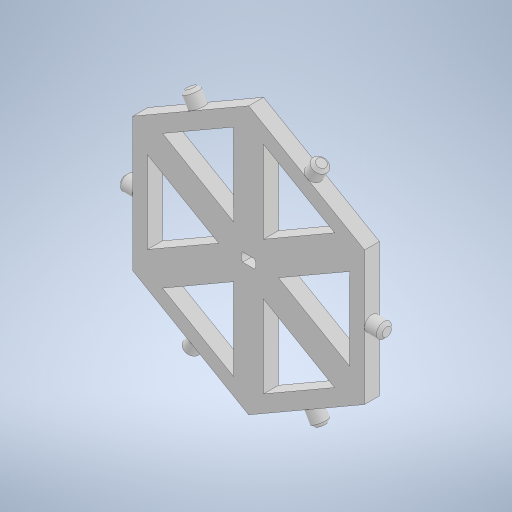
# Autodesk Inventor part: inner_case_bottom
Saved by Autodesk Inventor 2024 (Build 280153000, 153)
## iProperties
Created: 2024-03-18
Part Number: inner_case_bottom
Material: 일반
Document SubType Name: Modeling
Designer: SSAFY
Density: 1 g/cm^3
Appearance: 기본값
Author: SSAFY
Autodesk Inventor part; units mm, degrees
ref_plane "YZ Plane" through (0, 0, 0) normal (1, 0, 0) x (0, 1, 0)
ref_plane "XZ Plane" through (0, 0, 0) normal (0, 1, 0) x (-1, 0, 0)
ref_plane "XY Plane" through (0, 0, 0) normal (0, 0, 1) x (1, 0, 0)
sketch "스케치1" plane through (0, 0, 0) normal (0, 0, 1) x (1, 0, 0)
  line L0 (0.041, 45.0463) -> (39.005, 22.534)
  line L1 (39.005, 22.534) -> (38.9908, -22.466)
  line L2 (38.9908, -22.466) -> (0.0125, -44.9537)
  line L3 (0.0125, -44.9537) -> (-38.9515, -22.4414)
  line L4 (-38.9515, -22.4414) -> (-38.9373, 22.5586)
  line L5 (-38.9373, 22.5586) -> (0.041, 45.0463)
  line L6 (-38.9373, 22.5586) -> (0, 0)
  line L7 (0, 0) -> (-0.0392, 45.0926)
  line L8 (-5.0075, 8.6797) -> (-5.0316, 36.3473)
  line L9 (0.0143, -39.1802) -> (0.0341, -39.1916)
  line L10 (-28.9475, 22.5495) -> (-5.0075, 8.6797)
  line L11 (-28.9475, 22.5495) -> (-5.0316, 36.3473)
  line L12 (-0.0341, 39.2305) -> (0.0392, 39.2728)
  line L13 (5.0131, 8.6765) -> (28.9619, 22.5311)
  line L14 (5.0547, 36.3441) -> (28.9619, 22.5311)
  line L15 (5.0547, 36.3441) -> (5.0131, 8.6765)
  line L16 (10.0206, -0.0032) -> (33.9935, -13.8162)
  line L17 (34.0023, 13.7945) -> (33.9935, -13.8162)
  line L18 (34.0023, 13.7945) -> (10.0206, -0.0032)
  line L19 (5.0075, -8.6797) -> (5.0316, -36.3473)
  line L20 (28.9475, -22.5495) -> (5.0316, -36.3473)
  line L21 (28.9475, -22.5495) -> (5.0075, -8.6797)
  line L22 (-5.0131, -8.6765) -> (-28.9619, -22.5311)
  line L23 (-5.0547, -36.3441) -> (-28.9619, -22.5311)
  line L24 (-5.0547, -36.3441) -> (-5.0131, -8.6765)
  line L25 (-10.0206, 0.0032) -> (-33.9935, 13.8162)
  line L26 (-34.0023, -13.7945) -> (-33.9935, 13.8162)
  line L27 (-34.0023, -13.7945) -> (-10.0206, 0.0032)
  circle A0 centre (0, 0) radius 2.5
  line L28 (-2.0013, 1.4983) -> (1.9987, 1.5017)
  line L29 (-1.9987, -1.5017) -> (2.0013, -1.4983)
  dimension "d19" = 45
  dimension "d20" = 5
  dimension "d22" = 5
  dimension "d23" = 5
  dimension "d26" = 360
  dimension "d28" = 5
  dimension "d29" = 1.5
  dimension "d30" = 1.5
  constraints: 60 end point, 4 coincident, 4 point on circle, 3 point on line, 1 centre point, 1 parallel, 1 perpendicular, 41 other
  measures "d19" distance of L3.end L4.end
  measures "d20" distance between parallel lines of L7 L8
  measures "d22" distance between parallel lines of L11 L5
  measures "d23" distance between parallel lines of L6 L10
  measures "d28" diameter of A0
  measures "d29" distance from line of L28 L6.end
  measures "d30" distance from line of L29 point (0, 0)
extrude "돌출1" add sketch "스케치1" along normal blind 5 contours L0 L1 L2 L3 L4 L6 A0 L7 L5 | L7 A0 L6 L5 | A0 L28 L7 | L7 L28 A0 | L29 A0
sketch "스케치2" plane through (0.041, 45.0463, 5) normal (0.5002744, 0.8658669, 0) x (0.8658669, -0.5002744, 0)
  line L0 (45, 5) -> (0, 5) construction
  circle A0 centre (22.5, 2.5) radius 2.5
  point P0 (22.5, 5)
  point P1 (22.5, 5)
  dimension "d31" = 5
  dimension "d32" = 0
  constraints: 1 centre point, 1 midpoint, 1 tangent
  measures "d31" diameter of A0
  measures "d32" horizontal distance of point (22.5, 5) A0.centre
extrude "돌출2" add sketch "스케치2" along normal blind 5
chamfer "모따기1" distance 1 angle 45 1 edges at (19.8597, 39.3701, 2.5)
pattern_circular "원형 패턴1" count 6 over 360 about axis through (0, 0, -10) along (0, 0, 1) of "돌출2", "모따기1"
